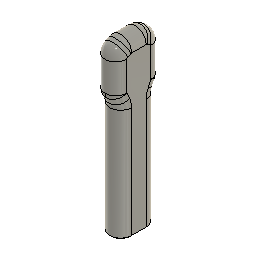
Prolunga_freni_rev_1.1 (Autodesk Fusion 360 design; units mm, degrees)
Autodesk Fusion 360 part; units mm, degrees
sketch "Schizzo1" plane through (0, 0, 0) normal (1, 0, 0) x (0, 1, 0)
  line L0 (18.245, 0) -> (18.245, 111.7185)
  line L1 (19.2011, 116.0715) -> (22.0439, 122.231)
  line L2 (23, 126.584) -> (23, 156.0021)
  line L3 (15.7382, 167.3516) -> (12.4928, 168.8495)
  line L4 (7.2545, 170) -> (0, 170)
  line L5 (18.245, 0) -> (0, 0)
  line L6 (0, 0) -> (0, 170) construction
  arc A0 (12.4928, 168.8495) -> (7.2545, 170) centre (7.2545, 157.5) ccw
  arc A1 (23, 156.0021) -> (15.7382, 167.3516) centre (10.5, 156.0021) ccw
  arc A2 (22.0439, 122.231) -> (23, 126.584) centre (12.6125, 126.584) ccw
  arc A3 (19.2011, 116.0715) -> (18.245, 111.7185) centre (28.6325, 111.7185) ccw
  line L7 (-18.245, 0) -> (0, 0)
  arc A4 (-18.245, 111.7185) -> (-19.2011, 116.0715) centre (-28.6325, 111.7185) ccw
  line L8 (-19.2011, 116.0715) -> (-22.0439, 122.231)
  arc A5 (-23, 126.584) -> (-22.0439, 122.231) centre (-12.6125, 126.584) ccw
  line L9 (-23, 126.584) -> (-23, 156.0021)
  arc A6 (-15.7382, 167.3516) -> (-23, 156.0021) centre (-10.5, 156.0021) ccw
  line L10 (-15.7382, 167.3516) -> (-12.4928, 168.8495)
  arc A7 (-7.2545, 170) -> (-12.4928, 168.8495) centre (-7.2545, 157.5) ccw
  line L11 (-7.2545, 170) -> (0, 170)
  line L12 (-18.245, 0) -> (-18.245, 111.7185)
  line L13 (-8.245, 0) -> (-8.245, 50)
  line L14 (-8.245, 50) -> (8.245, 50)
  line L15 (8.245, 50) -> (8.245, 0)
  point P0 (18.245, 114)
  point P1 (23, 124.3025)
  point P2 (23, 164)
  point P3 (10, 170)
  point P4 (0, 50)
  dimension "d1" = 170
  dimension "d2" = 18.245
  dimension "d3" = 56
  dimension "d4" = 10
  dimension "d5" = 23
  dimension "d6" = 23
  dimension "d7" = 6
  dimension "d8" = 12.5
  dimension "d9" = 12.5
  dimension "d10" = 10.3875
  dimension "d16" = 50
  dimension "d17" = 16.49
  constraint vertical L0
  constraint perpendicular L1 L3
  constraint horizontal L4
  constraint coincident L5.end L6.start
  constraint perpendicular L0 L5
  constraint vertical L6
  constraint coincident P3 L3
  constraint coincident P3 L4
  constraint tangent L3 A0
  constraint tangent L4 A0
  constraint coincident P2 L2
  constraint coincident P2 L3
  constraint tangent L2 A1
  constraint tangent L3 A1
  constraint coincident P1 L1
  constraint coincident P1 L2
  constraint tangent L1 A2
  constraint tangent L2 A2
  constraint coincident P0 L0
  constraint coincident P0 L1
  constraint tangent L0 A3
  constraint tangent L1 A3
  constraint equal A2 A3
  constraint symmetric L0.start L6 L7.start
  constraint symmetric L4.end L6 L11.end
  constraint symmetric L5.end L6 L7.end
  constraint symmetric L6 L3.end L10.end
  constraint symmetric L6 L4.start A7.start
  constraint symmetric L6 A0 A7
  constraint symmetric L6 L2.end L9.end
  constraint symmetric L6 L3.start A6.start
  constraint symmetric L6 A1 A6
  constraint symmetric L6 L1.end L8.end
  constraint symmetric L6 L2.start A5.start
  constraint symmetric L6 A2 A5
  constraint symmetric L6 L0.end A4.start
  constraint symmetric L6 L1.start A4.end
  constraint symmetric L6 A3 A4
  constraint coincident L7 L13.start
  constraint perpendicular L7 L13
  constraint perpendicular L6 L14
  constraint coincident L5 L15.end
  constraint perpendicular L5 L15
  constraint coincident L14 P4
  constraint midpoint L14 P4
  constraint coincident L6 P4
  measures "d1" distance of L4 L5
  measures "d2" distance of L0 L6
  measures "d3" distance of P0 L4
  measures "d4" distance of P3 L4.end
  measures "d5" distance of P1 L6
  measures "d6" distance of P2 L6
  measures "d7" distance of P2 L4
  measures "d8" radius of A0
  measures "d9" radius of A1
  measures "d10" radius of A2
  measures "d16" distance of L13.start L13.end
  measures "d17" distance of L13 L15
extrude "Estrusione1" add sketch "Schizzo1" along normal mid plane 21.84
extrude "Estrusione2" cut sketch "Schizzo1" along normal mid plane 7.09 contours L5 L7 L13 L14 L15
fillet "Raccordo1" radius 10.92 34 edges at (-10.92, -18.245, 55.8593) (-10.92, -18.4868, 113.9469) (-10.92, -20.6225, 119.1512) (-10.92, -22.7582, 124.3556) (-10.92, -23, 141.293) (-10.92, -21.0292, 162.739) (-10.92, -14.1155, 168.1005) (-10.92, -9.9361, 169.709) (-10.92, 0, 170) (-10.92, 9.9361, 169.709) (-10.92, 14.1155, 168.1005) (-10.92, 21.0292, 162.739) (-10.92, 23, 141.293) (-10.92, 22.7582, 124.3556) (-10.92, 20.6225, 119.1512) (-10.92, 18.4868, 113.9469) (-10.92, 18.245, 55.8593) (10.92, 18.245, 55.8593) (10.92, 18.4868, 113.9469) (10.92, 20.6225, 119.1512) (10.92, 22.7582, 124.3556) (10.92, 23, 141.293) (10.92, 21.0292, 162.739) (10.92, 14.1155, 168.1005) (10.92, 9.9361, 169.709) (10.92, 0, 170) (10.92, -9.9361, 169.709) (10.92, -14.1155, 168.1005) (10.92, -21.0292, 162.739) (10.92, -23, 141.293) (10.92, -22.7582, 124.3556) (10.92, -20.6225, 119.1512) (10.92, -18.4868, 113.9469) (10.92, -18.245, 55.8593)
chamfer "Smusso1" distance 1 angle 45 4 edges at (-3.545, 0, 0) (0, 8.245, 0) (3.545, 0, 0) (0, -8.245, 0)
chamfer "Smusso1" distance 1 angle 45 4 edges at (0, -18.245, 0) (10.92, 0, 0) (0, 18.245, 0) (-10.92, 0, 0)
equation "d1 = lunghezza_prolunga_freno"
equation "d2 = d17 / 2 + 10 mm"
equation "d5 = d6"
equation "d10 = -d2 * 2.5 + 56 mm"
equation "offset_incastro = 0.25 mm" comment "Modificare questo valore per permettere l'incastro perfetto. (Valore di default 0.25 mm)"
equation "larghezza_incastro = 16.24 mm" comment "Modificare questo valore per allargare o diminuire la larghezza dell'incastro del freno. (Valore di default 16.24 mm)"
equation "spessore_incastro = 6.84 mm" comment "Modificare questo valore per allargare o diminuire lo spessore dell'incastro del freno. (Valore di default 4.1 mm)"
equation "profondita_incastro = 50 mm" comment "Modificare questo valore per allargare o diminuire la profondità dell'incastro del freno. (Valore di default 50 mm)"
equation "lunghezza_prolunga_freno = 170 mm" comment "Modificare questo valore per allungare o accorciare la prolunga del freno. (Valore di default 170 mm)"
equation "d16 = profondita_incastro"
equation "d17 = larghezza_incastro + offset_incastro"
equation "d18 = spessore_incastro + 15 mm"
equation "d20 = spessore_incastro + offset_incastro"
equation "d23 = d18 / 2"
named bodies: "prolunga_freno"
